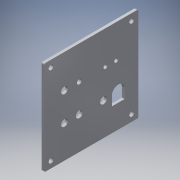
# Autodesk Inventor part: PP-LAS-0001
Saved by Autodesk Inventor 2018.3 (Build 223284000, 284)
## iProperties
Created: 2021-05-05
Part Number: PP-LAS-0001
Material: Plástico ABS
Document SubType Name: Modeling
Designer: L.Aguerre
Density: 1.06 g/cm^3
Appearance: Suave - Blanco
Description: FRENTE DE PANEL SERIGRAFIADO
Author: laguerre
Autodesk Inventor part; units mm, degrees
(part 1 of 3)
ref_plane "YZ Plane" through (0, 0, 0) normal (1, 0, 0) x (0, 1, 0)
ref_plane "XZ Plane" through (0, 0, 0) normal (0, 1, 0) x (-1, 0, 0)
ref_plane "XY Plane" through (0, 0, 0) normal (0, 0, 1) x (1, 0, 0)
sketch "Boceto39" plane through (0, 0, 0) normal (0, 0, 1) x (1, 0, 0)
  line L0 (-34, 35) -> (34, 35)
  line L1 (35, 34) -> (35, -34)
  line L2 (34, -35) -> (-34, -35)
  line L3 (-35, -34) -> (-35, 34)
  arc A0 (-34, 35) -> (-35, 34) centre (-34, 34) ccw
  arc A1 (35, 34) -> (34, 35) centre (34, 34) ccw
  arc A2 (34, -35) -> (35, -34) centre (34, -34) ccw
  arc A3 (-35, -34) -> (-34, -35) centre (-34, -34) ccw
  point P0 (0, 0)
  point P1 (0, 35)
  point P2 (-35, 0)
  dimension "d373" = 70
  dimension "d374" = 70
  dimension "d375" = 1
  constraints: 8 end point, 8 point on circle, 8 tangent, 4 centre point, 3 equal radius, 2 midpoint, 2 parallel, 1 horizontal, 1 horizontal alignment, 1 perpendicular, 1 vertical alignment
  measures "d373" distance between parallel lines of L1 L3
  measures "d374" distance between parallel lines of L2 L0
  measures "d375" radius of A0
extrude "Extrusión13" add sketch "Boceto39" along normal blind 2
sketch "Boceto43" plane through (0, 0, 2) normal (0, 0, 1) x (1, 0, 0)
  line L0 (-30, 30) -> (30, 30) construction
  line L1 (30, 30) -> (30, -30) construction
  line L2 (30, -30) -> (-30, -30) construction
  line L3 (-30, -30) -> (-30, 30) construction
  point P0 (0, 0)
  point P1 (0, 30)
  point P2 (-30, 0)
  dimension "d402" = 60
  constraints: 8 end point, 2 coincident, 2 midpoint, 2 parallel, 2 perpendicular, 1 horizontal, 1 horizontal alignment, 1 point on line, 1 vertical alignment
  measures "d402" distance of L0.start L0.end
hole "Agujero2" at (30, 30, 2) at (30, -30, 2) at (-30, -30, 2) at (-30, 30, 2) direction (0, 0, -1) diameter 3.5 depth 8 tip angle 118
sketch "Boceto40" plane through (0, 0, 2) normal (0, 0, 1) x (1, 0, 0)
  line L0 (-25, 0) -> (-4, 0)
  line L1 (-2, -2) -> (-2, -18)
  line L2 (-4, -20) -> (-25, -20)
  line L3 (-27, -18) -> (-27, -2)
  line L4 (4, 0) -> (25, 0)
  line L5 (27, -2) -> (27, -18)
  line L6 (25, -20) -> (4, -20)
  line L7 (2, -18) -> (2, -2)
  line L8 (-25, 20) -> (25, 20)
  line L9 (27, 18) -> (27, 5)
  line L10 (25, 3) -> (-25, 3)
  line L11 (-27, 5) -> (-27, 18)
  arc A0 (-27, -18) -> (-25, -20) centre (-25, -18) ccw
  arc A1 (-4, -20) -> (-2, -18) centre (-4, -18) ccw
  arc A2 (-2, -2) -> (-4, 0) centre (-4, -2) ccw
  arc A3 (-25, 0) -> (-27, -2) centre (-25, -2) ccw
  arc A4 (4, 0) -> (2, -2) centre (4, -2) ccw
  arc A5 (2, -18) -> (4, -20) centre (4, -18) ccw
  arc A6 (25, -20) -> (27, -18) centre (25, -18) ccw
  arc A7 (27, -2) -> (25, 0) centre (25, -2) ccw
  line L12 (-34, -35) -> (34, -35) projected
  arc A8 (-27, 5) -> (-25, 3) centre (-25, 5) ccw
  arc A9 (-25, 20) -> (-27, 18) centre (-25, 18) ccw
  arc A10 (27, 18) -> (25, 20) centre (25, 18) ccw
  arc A11 (25, 3) -> (27, 5) centre (25, 5) ccw
  line L13 (25, 19.7) -> (-25, 19.7)
  arc A12 (-25, 19.7) -> (-26.7, 18) centre (-25, 18) ccw
  line L14 (-26.7, 18) -> (-26.7, 5)
  arc A13 (-26.7, 5) -> (-25, 3.3) centre (-25, 5) ccw
  line L15 (-25, 3.3) -> (25, 3.3)
  arc A14 (25, 3.3) -> (26.7, 5) centre (25, 5) ccw
  line L16 (26.7, 5) -> (26.7, 18)
  arc A15 (26.7, 18) -> (25, 19.7) centre (25, 18) ccw
  line L17 (-4, -0.3) -> (-25, -0.3)
  arc A16 (-25, -0.3) -> (-26.7, -2) centre (-25, -2) ccw
  line L18 (-26.7, -2) -> (-26.7, -18)
  arc A17 (-26.7, -18) -> (-25, -19.7) centre (-25, -18) ccw
  line L19 (-25, -19.7) -> (-4, -19.7)
  arc A18 (-4, -19.7) -> (-2.3, -18) centre (-4, -18) ccw
  line L20 (-2.3, -18) -> (-2.3, -2)
  arc A19 (-2.3, -2) -> (-4, -0.3) centre (-4, -2) ccw
  line L21 (25, -0.3) -> (4, -0.3)
  arc A20 (4, -0.3) -> (2.3, -2) centre (4, -2) ccw
  line L22 (2.3, -2) -> (2.3, -18)
  arc A21 (2.3, -18) -> (4, -19.7) centre (4, -18) ccw
  line L23 (4, -19.7) -> (25, -19.7)
  arc A22 (25, -19.7) -> (26.7, -18) centre (25, -18) ccw
  line L24 (26.7, -18) -> (26.7, -2)
  arc A23 (26.7, -2) -> (25, -0.3) centre (25, -2) ccw
  point P0 (0, 0)
  point P1 (-27, 0)
  point P2 (-2, -20)
  point P3 (-27, -20)
  point P4 (27, -20)
  point P5 (2, -20)
  point P6 (0, 20)
  dimension "d378" = 2
  dimension "d379" = 2
  dimension "d380" = 25
  dimension "d381" = 25
  dimension "d382" = 20
  dimension "d383" = 2
  dimension "d385" = 3
  dimension "d386" = 2
  dimension "d387" = 17
  dimension "d388" = 0.3
  dimension "d389" = 0.3
  dimension "d390" = 0.3
  dimension "d477" = 20
  constraints: 48 end point, 48 point on circle, 24 centre point, 24 tangent, 12 parallel, 10 equal radius, 10 point on line, 6 perpendicular, 3 collinear, 3 horizontal, 1 midpoint, 1 vertical alignment, 21 other
  measures "d378" distance from line of point (0, 0) L1
  measures "d379" distance from line of point (0, 0) L7
  measures "d380" distance of point (-2, -20) point (-27, -20)
  measures "d381" distance of point (27, -20) point (2, -20)
  measures "d382" distance of point (-27, -20) point (-27, 0)
  measures "d383" radius of A0
  measures "d385" distance between parallel lines of L10 L0
  measures "d386" radius of A8
  measures "d387" distance between parallel lines of L8 L10
  measures "d388" distance between parallel lines of L15 L10
  measures "d389" distance between parallel lines of L4 L21
  measures "d390" distance between parallel lines of L0 L17
  measures "d477" distance from line of L6 point (0, 0)
extrude "Extrusión14" add sketch "Boceto40" along normal blind 0.001
sketch "Boceto41" plane through (0, 0, 2) normal (0, 0, 1) x (1, 0, 0)
  circle A0 centre (-20, -10.7) radius 5 construction
  line L0 (-34, -35) -> (34, -35) projected
  line L1 (-35, 34) -> (-35, -34) projected
  circle A1 centre (-9, -10.7) radius 2.5
  line L2 (-20, -10.7) -> (-9, -10.7) construction
  line L3 (-4, -19.7) -> (-25, -19.7) projected
  circle A2 centre (9, -10.7) radius 2.5
  circle A3 centre (20, -10.7) radius 2.5
  line L4 (25, -19.7) -> (4, -19.7) projected
  circle A4 centre (-18.5, 10.3) radius 1.5
  circle A5 centre (-10.5, 10.3) radius 1.5
  line L5 (-18.5, 10.3) -> (-10.5, 10.3) construction
  line L6 (25, 3.3) -> (-25, 3.3) projected
  circle A6 centre (20, 10.3) radius 2.5
  circle A7 centre (9, 10.3) radius 1.75
  line L7 (9, -10.7) -> (20, -10.7) construction
  line L8 (9, 10.3) -> (20, 10.3) construction
  line L9 (-24.7, -10.7) -> (-24.7, -17.7)
  line L10 (-24.7, -17.7) -> (-15.3, -17.7)
  line L11 (-15.3, -17.7) -> (-15.3, -10.7)
  arc A8 (-15.3, -10.7) -> (-24.7, -10.7) centre (-20, -10.7) ccw
  line L12 (-20, -6) -> (-22.9713, -6) construction
  point P0 (0, 0)
  point P1 (-14.5, -10.7)
  point P2 (-14.5, -19.7)
  point P3 (-14.5, 10.3)
  point P4 (14.5, -10.7)
  point P5 (14.5, -19.7)
  point P6 (14.5, 10.3)
  point P7 (-20, -17.7)
  dimension "d393" = 10
  dimension "d396" = 5
  dimension "d397" = 11
  dimension "d399" = 11
  dimension "d410" = 9
  dimension "d415" = 3
  dimension "d416" = 7
  dimension "d417" = 8
  dimension "d418" = 3.5
  dimension "d419" = 11
  dimension "d474" = 9.4
  dimension "d475" = 7
  dimension "d476" = 4.7
  constraints: 16 end point, 9 centre point, 7 midpoint, 5 horizontal, 5 horizontal alignment, 5 vertical alignment, 4 equal radius, 3 point on circle, 3 tangent, 2 perpendicular, 1 coincident, 1 vertical
  measures "d393" diameter of A0
  measures "d396" diameter of A1
  measures "d397" distance of L2.start L2.end
  measures "d399" distance of L7.end L7.start
  measures "d410" distance between parallel lines of L2 L3
  measures "d415" diameter of A5
  measures "d416" distance between parallel lines of L5 L6
  measures "d417" distance of L5.start L5.end
  measures "d418" diameter of A7
  measures "d419" distance of L8.end L8.start
  measures "d474" distance of L9.end L10.end
  measures "d475" distance from line of L2.start L10
  measures "d476" distance from line of L2.start L12
extrude "Extrusión15" cut sketch "Boceto41" against normal blind 2
sketch "Boceto42" plane through (0, 0, 2) normal (0, 0, 1) x (1, 0, 0)
  line L0 (-19.9009, -2.7) -> (-1.3327, -2.7) construction
  line L1 (-1.3327, -2.7) -> (-1.3327, -6.6561) construction
  line L2 (-1.3327, -6.6561) -> (-19.9009, -6.6561) construction
  line L3 (-19.9009, -6.6561) -> (-19.9009, -2.7) construction
  line L4 (-11.8025, -15.7) -> (-8.1255, -15.7) construction
  line L5 (-8.1255, -15.7) -> (-8.1255, -16.9024) construction
  line L6 (-8.1255, -16.9024) -> (-11.8025, -16.9024) construction
  line L7 (-11.8025, -16.9024) -> (-11.8025, -15.7) construction
  line L8 (6.4191, -2.7) -> (25.511, -2.7) construction
  line L9 (25.511, -2.7) -> (25.511, -5.9558) construction
  line L10 (25.511, -5.9558) -> (6.4191, -5.9558) construction
  line L11 (6.4191, -5.9558) -> (6.4191, -2.7) construction
  line L12 (7.0108, -15.7) -> (12.5482, -15.7) construction
  line L13 (12.5482, -15.7) -> (12.5482, -16.8686) construction
  line L14 (12.5482, -16.8686) -> (7.0108, -16.8686) construction
  line L15 (7.0108, -16.8686) -> (7.0108, -15.7) construction
  line L16 (17.6981, -15.7) -> (23.2355, -15.7) construction
  line L17 (23.2355, -15.7) -> (23.2355, -15.9466) construction
  line L18 (23.2355, -15.9466) -> (17.6981, -15.9466) construction
  line L19 (17.6981, -15.9466) -> (17.6981, -15.7) construction
  circle A0 centre (9, -10.7) radius 2.5 projected
  line L20 (-18.1999, 5.1784) -> (-18.1999, 6.3) construction
  line L21 (-18.1999, 6.3) -> (-6.5736, 6.3) construction
  line L22 (-6.5736, 6.3) -> (-6.5736, 5.1784) construction
  line L23 (-6.5736, 5.1784) -> (-18.1999, 5.1784) construction
  line L24 (6.4525, 5.7678) -> (6.4525, 6.3) construction
  line L25 (6.4525, 6.3) -> (10.1295, 6.3) construction
  line L26 (10.1295, 6.3) -> (10.1295, 5.7678) construction
  line L27 (10.1295, 5.7678) -> (6.4525, 5.7678) construction
  circle A1 centre (-18.5, 10.3) radius 1.5 projected
  line L28 (-22.5122, 16.6992) -> (-6.3487, 16.6992) construction
  line L29 (-6.3487, 16.6992) -> (-6.3487, 14.435) construction
  line L30 (-6.3487, 14.435) -> (-22.5122, 14.435) construction
  line L31 (-22.5122, 14.435) -> (-22.5122, 16.6992) construction
  line L32 (6.7652, 14.2645) -> (6.7652, 16.6992) construction
  line L33 (6.7652, 16.6992) -> (24.191, 16.6992) construction
  line L34 (24.191, 16.6992) -> (24.191, 14.2645) construction
  line L35 (24.191, 14.2645) -> (6.7652, 14.2645) construction
  line L36 (17.5924, 5.1479) -> (17.5924, 6.3) construction
  line L37 (17.5924, 6.3) -> (21.2695, 6.3) construction
  line L38 (21.2695, 6.3) -> (21.2695, 5.1479) construction
  line L39 (21.2695, 5.1479) -> (17.5924, 5.1479) construction
  line L40 (-19.0013, -4.7421) -> (-19.7761, -4.7421)
  line L41 (-19.7761, -4.7421) -> (-19.7761, -4.5379)
  line L42 (-19.7761, -4.5379) -> (-19.5216, -4.5379)
  line L43 (-19.5216, -4.5379) -> (-19.5216, -2.9464)
  line L44 (-19.5216, -2.9464) -> (-19.7761, -2.9464)
  line L45 (-19.7761, -2.9464) -> (-19.7761, -2.7421)
  line L46 (-19.7761, -2.7421) -> (-19.0013, -2.7421)
  line L47 (-19.0013, -2.7421) -> (-19.0013, -2.9464)
  line L48 (-19.0013, -2.9464) -> (-19.2558, -2.9464)
  line L49 (-19.2558, -2.9464) -> (-19.2558, -4.5379)
  line L50 (-19.2558, -4.5379) -> (-19.0013, -4.5379)
  line L51 (-19.0013, -4.5379) -> (-19.0013, -4.7421)
  line L52 (-17.2412, -4.7421) -> (-17.5394, -4.7421)
  line L53 (-17.5394, -4.7421) -> (-18.4244, -3.0177)
  line L54 (-18.4244, -3.0177) -> (-18.4244, -4.7421)
  line L55 (-18.4244, -4.7421) -> (-18.6723, -4.7421)
  line L56 (-18.6723, -4.7421) -> (-18.6723, -2.7421)
  line L57 (-18.6723, -2.7421) -> (-18.2947, -2.7421)
  line L58 (-18.2947, -2.7421) -> (-17.4892, -4.3256)
  line L59 (-17.4892, -4.3256) -> (-17.4892, -2.7421)
  line L60 (-17.4892, -2.7421) -> (-17.2412, -2.7421)
  line L61 (-17.2412, -2.7421) -> (-17.2412, -4.7421)
  spline S0 degree 2 poles (-15.5719, -3.3451) (-15.5719, -3.4747) (-15.6642, -3.7081) (-15.7469, -3.7891) knots 0 0 0 1 2 2 2
  spline S1 degree 2 poles (-15.7469, -3.7891) (-15.8506, -3.8912) (-16.131, -3.9966) (-16.3449, -3.9966) knots 0 0 0 1 2 2 2
  line L62 (-16.3449, -3.9966) -> (-16.5702, -3.9966)
  line L63 (-16.5702, -3.9966) -> (-16.5702, -4.7421)
  line L64 (-16.5702, -4.7421) -> (-16.836, -4.7421)
  line L65 (-16.836, -4.7421) -> (-16.836, -2.7421)
  line L66 (-16.836, -2.7421) -> (-16.3336, -2.7421)
  spline S2 degree 2 poles (-16.3336, -2.7421) (-16.1553, -2.7421) (-15.9057, -2.8005) (-15.8101, -2.8669) knots 0 0 0 1 2 2 2
  spline S3 degree 2 poles (-15.8101, -2.8669) (-15.6983, -2.9431) (-15.5719, -3.1781) (-15.5719, -3.3451) knots 0 0 0 1 2 2 2
  spline S4 degree 2 poles (-15.849, -3.3532) (-15.849, -3.2494) (-15.9203, -3.0971) (-15.9932, -3.0485) knots 0 0 0 1 2 2 2
  spline S5 degree 2 poles (-15.9932, -3.0485) (-16.0565, -3.0063) (-16.225, -2.9723) (-16.3498, -2.9723) knots 0 0 0 1 2 2 2
  line L67 (-16.3498, -2.9723) -> (-16.5702, -2.9723)
  line L68 (-16.5702, -2.9723) -> (-16.5702, -3.7697)
  line L69 (-16.5702, -3.7697) -> (-16.3887, -3.7697)
  spline S6 degree 2 poles (-16.3887, -3.7697) (-16.2266, -3.7697) (-16.0273, -3.7178) (-15.9625, -3.6498) knots 0 0 0 1 2 2 2
  spline S7 degree 2 poles (-15.9625, -3.6498) (-15.9025, -3.5898) (-15.849, -3.4488) (-15.849, -3.3532) knots 0 0 0 1 2 2 2
  spline S8 degree 2 poles (-14.6205, -4.7843) (-14.7971, -4.7843) (-15.0597, -4.6919) (-15.1521, -4.5995) knots 0 0 0 1 2 2 2
  spline S9 degree 2 poles (-15.1521, -4.5995) (-15.2574, -4.4958) (-15.3433, -4.2041) (-15.3433, -3.9901) knots 0 0 0 1 2 2 2
  line L70 (-15.3433, -3.9901) -> (-15.3433, -2.7421)
  line L71 (-15.3433, -2.7421) -> (-15.0775, -2.7421)
  line L72 (-15.0775, -2.7421) -> (-15.0775, -3.9901)
  spline S10 degree 2 poles (-15.0775, -3.9901) (-15.0775, -4.1295) (-15.0419, -4.3175) (-14.9916, -4.3937) knots 0 0 0 1 2 2 2
  spline S11 degree 2 poles (-14.9916, -4.3937) (-14.9381, -4.4747) (-14.7534, -4.5574) (-14.6205, -4.5574) knots 0 0 0 1 2 2 2
  spline S12 degree 2 poles (-14.6205, -4.5574) (-14.4957, -4.5574) (-14.3012, -4.4747) (-14.2477, -4.3937) knots 0 0 0 1 2 2 2
  spline S13 degree 2 poles (-14.2477, -4.3937) (-14.1975, -4.3175) (-14.1618, -4.1311) (-14.1618, -3.9966) knots 0 0 0 1 2 2 2
  line L73 (-14.1618, -3.9966) -> (-14.1618, -2.7421)
  line L74 (-14.1618, -2.7421) -> (-13.896, -2.7421)
  line L75 (-13.896, -2.7421) -> (-13.896, -3.9901)
  spline S14 degree 2 poles (-13.896, -3.9901) (-13.896, -4.1992) (-13.9803, -4.4974) (-14.0872, -4.5995) knots 0 0 0 1 2 2 2
  spline S15 degree 2 poles (-14.0872, -4.5995) (-14.1829, -4.6935) (-14.4357, -4.7843) (-14.6205, -4.7843) knots 0 0 0 1 2 2 2
  line L76 (-13.0484, -4.7421) -> (-13.0484, -2.9788)
  line L77 (-13.0484, -2.9788) -> (-13.7193, -2.9788)
  line L78 (-13.7193, -2.9788) -> (-13.7193, -2.7421)
  line L79 (-13.7193, -2.7421) -> (-12.1116, -2.7421)
  line L80 (-12.1116, -2.7421) -> (-12.1116, -2.9788)
  line L81 (-12.1116, -2.9788) -> (-12.7825, -2.9788)
  line L82 (-12.7825, -2.9788) -> (-12.7825, -4.7421)
  line L83 (-12.7825, -4.7421) -> (-13.0484, -4.7421)
  line L84 (-9.9738, -4.7421) -> (-10.9495, -4.7421)
  line L85 (-10.9495, -4.7421) -> (-10.9495, -4.5379)
  line L86 (-10.9495, -4.5379) -> (-10.5864, -4.5379)
  line L87 (-10.5864, -4.5379) -> (-10.5864, -3.1976)
  line L88 (-10.5864, -3.1976) -> (-10.9495, -3.1976)
  line L89 (-10.9495, -3.1976) -> (-10.9495, -3.0144)
  spline S16 degree 2 poles (-10.9495, -3.0144) (-10.7436, -3.0144) (-10.5492, -2.8977) (-10.5362, -2.7357) knots 0 0 0 1 2 2 2
  line L90 (-10.5362, -2.7357) -> (-10.3287, -2.7357)
  line L91 (-10.3287, -2.7357) -> (-10.3287, -4.5379)
  line L92 (-10.3287, -4.5379) -> (-9.9738, -4.5379)
  line L93 (-9.9738, -4.5379) -> (-9.9738, -4.7421)
  line L94 (-8.3725, -4.7421) -> (-9.6059, -4.7421)
  line L95 (-9.6059, -4.7421) -> (-9.6059, -4.4585)
  spline S17 degree 2 poles (-9.6059, -4.4585) (-9.473, -4.3337) (-9.2364, -4.1019) (-9.1229, -3.9771) knots 0 0 0 1 2 2 2
  spline S18 degree 2 poles (-9.1229, -3.9771) (-8.8944, -3.7259) (-8.7274, -3.4245) (-8.7274, -3.264) knots 0 0 0 1 2 2 2
  spline S19 degree 2 poles (-8.7274, -3.264) (-8.7274, -3.1797) (-8.7793, -3.0533) (-8.8263, -3.0128) knots 0 0 0 1 2 2 2
  spline S20 degree 2 poles (-8.8263, -3.0128) (-8.8733, -2.9723) (-8.9965, -2.9318) (-9.071, -2.9318) knots 0 0 0 1 2 2 2
  spline S21 degree 2 poles (-9.071, -2.9318) (-9.1424, -2.9318) (-9.2882, -2.9674) (-9.3547, -2.995) knots 0 0 0 1 2 2 2
  spline S22 degree 2 poles (-9.3547, -2.995) (-9.4114, -3.0177) (-9.5167, -3.0825) (-9.5492, -3.1052) knots 0 0 0 1 2 2 2
  line L96 (-9.5492, -3.1052) -> (-9.5637, -3.1052)
  line L97 (-9.5637, -3.1052) -> (-9.5637, -2.8199)
  spline S23 degree 2 poles (-9.5637, -2.8199) (-9.4811, -2.7794) (-9.1845, -2.7) (-9.0516, -2.7) knots 0 0 0 1 2 2 2
  spline S24 degree 2 poles (-9.0516, -2.7) (-8.7712, -2.7) (-8.4552, -2.9966) (-8.4552, -3.2494) knots 0 0 0 1 2 2 2
  spline S25 degree 2 poles (-8.4552, -3.2494) (-8.4552, -3.3677) (-8.5103, -3.5655) (-8.5589, -3.6498) knots 0 0 0 1 2 2 2
  spline S26 degree 2 poles (-8.5589, -3.6498) (-8.6075, -3.7373) (-8.7485, -3.9091) (-8.8263, -3.9917) knots 0 0 0 1 2 2 2
  spline S27 degree 2 poles (-8.8263, -3.9917) (-8.9527, -4.1295) (-9.2623, -4.4245) (-9.3547, -4.5104) knots 0 0 0 1 2 2 2
  line L98 (-9.3547, -4.5104) -> (-8.3725, -4.5104)
  line L99 (-8.3725, -4.5104) -> (-8.3725, -4.7421)
  line L100 (-6.5978, -2.7421) -> (-7.2866, -4.7421)
  line L101 (-7.2866, -4.7421) -> (-7.5735, -4.7421)
  line L102 (-7.5735, -4.7421) -> (-8.2623, -2.7421)
  line L103 (-8.2623, -2.7421) -> (-7.977, -2.7421)
  line L104 (-7.977, -2.7421) -> (-7.4227, -4.4034)
  line L105 (-7.4227, -4.4034) -> (-6.8684, -2.7421)
  line L106 (-6.8684, -2.7421) -> (-6.5978, -2.7421)
  spline S28 degree 2 poles (-10.7025, -16.1789) (-10.7025, -16.2762) (-10.7717, -16.4512) (-10.8337, -16.512) knots 0 0 0 1 2 2 2
  spline S29 degree 2 poles (-10.8337, -16.512) (-10.9115, -16.5886) (-11.1218, -16.6676) (-11.2823, -16.6676) knots 0 0 0 1 2 2 2
  line L107 (-11.2823, -16.6676) -> (-11.4512, -16.6676)
  line L108 (-11.4512, -16.6676) -> (-11.4512, -17.2267)
  line L109 (-11.4512, -17.2267) -> (-11.6506, -17.2267)
  line L110 (-11.6506, -17.2267) -> (-11.6506, -15.7267)
  line L111 (-11.6506, -15.7267) -> (-11.2738, -15.7267)
  spline S30 degree 2 poles (-11.2738, -15.7267) (-11.1401, -15.7267) (-10.9529, -15.7705) (-10.8811, -15.8203) knots 0 0 0 1 2 2 2
  spline S31 degree 2 poles (-10.8811, -15.8203) (-10.7973, -15.8775) (-10.7025, -16.0537) (-10.7025, -16.1789) knots 0 0 0 1 2 2 2
  spline S32 degree 2 poles (-10.9103, -16.185) (-10.9103, -16.1072) (-10.9638, -15.9929) (-11.0185, -15.9565) knots 0 0 0 1 2 2 2
  spline S33 degree 2 poles (-11.0185, -15.9565) (-11.0659, -15.9249) (-11.1923, -15.8994) (-11.2859, -15.8994) knots 0 0 0 1 2 2 2
  line L112 (-11.2859, -15.8994) -> (-11.4512, -15.8994)
  line L113 (-11.4512, -15.8994) -> (-11.4512, -16.4974)
  line L114 (-11.4512, -16.4974) -> (-11.3151, -16.4974)
  spline S34 degree 2 poles (-11.3151, -16.4974) (-11.1935, -16.4974) (-11.044, -16.4585) (-10.9954, -16.4075) knots 0 0 0 1 2 2 2
  spline S35 degree 2 poles (-10.9954, -16.4075) (-10.9504, -16.3625) (-10.9103, -16.2567) (-10.9103, -16.185) knots 0 0 0 1 2 2 2
  line L115 (-9.6437, -17.2267) -> (-10.5128, -17.2267)
  line L116 (-10.5128, -17.2267) -> (-10.5128, -15.7267)
  line L117 (-10.5128, -15.7267) -> (-10.3135, -15.7267)
  line L118 (-10.3135, -15.7267) -> (-10.3135, -17.0493)
  line L119 (-10.3135, -17.0493) -> (-9.6437, -17.0493)
  line L120 (-9.6437, -17.0493) -> (-9.6437, -17.2267)
  spline S36 degree 2 poles (-8.963, -17.2583) (-9.0955, -17.2583) (-9.2924, -17.1891) (-9.3617, -17.1198) knots 0 0 0 1 2 2 2
  spline S37 degree 2 poles (-9.3617, -17.1198) (-9.4407, -17.042) (-9.5051, -16.8232) (-9.5051, -16.6627) knots 0 0 0 1 2 2 2
  line L121 (-9.5051, -16.6627) -> (-9.5051, -15.7267)
  line L122 (-9.5051, -15.7267) -> (-9.3058, -15.7267)
  line L123 (-9.3058, -15.7267) -> (-9.3058, -16.6627)
  spline S38 degree 2 poles (-9.3058, -16.6627) (-9.3058, -16.7673) (-9.279, -16.9083) (-9.2414, -16.9654) knots 0 0 0 1 2 2 2
  spline S39 degree 2 poles (-9.2414, -16.9654) (-9.2012, -17.0262) (-9.0627, -17.0882) (-8.963, -17.0882) knots 0 0 0 1 2 2 2
  spline S40 degree 2 poles (-8.963, -17.0882) (-8.8694, -17.0882) (-8.7235, -17.0262) (-8.6834, -16.9654) knots 0 0 0 1 2 2 2
  spline S41 degree 2 poles (-8.6834, -16.9654) (-8.6457, -16.9083) (-8.619, -16.7685) (-8.619, -16.6676) knots 0 0 0 1 2 2 2
  line L124 (-8.619, -16.6676) -> (-8.619, -15.7267)
  line L125 (-8.619, -15.7267) -> (-8.4196, -15.7267)
  line L126 (-8.4196, -15.7267) -> (-8.4196, -16.6627)
  spline S42 degree 2 poles (-8.4196, -16.6627) (-8.4196, -16.8195) (-8.4828, -17.0432) (-8.5631, -17.1198) knots 0 0 0 1 2 2 2
  spline S43 degree 2 poles (-8.5631, -17.1198) (-8.6348, -17.1903) (-8.8244, -17.2583) (-8.963, -17.2583) knots 0 0 0 1 2 2 2
  spline S44 degree 2 poles (-7.5055, -17.2559) (-7.6648, -17.2559) (-7.9285, -17.1587) (-8.0234, -17.0602) knots 0 0 0 1 2 2 2
  spline S45 degree 2 poles (-8.0234, -17.0602) (-8.1182, -16.9605) (-8.2191, -16.6664) (-8.2191, -16.4755) knots 0 0 0 1 2 2 2
  spline S46 degree 2 poles (-8.2191, -16.4755) (-8.2191, -16.2944) (-8.117, -16.0075) (-8.0221, -15.9054) knots 0 0 0 1 2 2 2
  spline S47 degree 2 poles (-8.0221, -15.9054) (-7.931, -15.807) (-7.6636, -15.7) (-7.5043, -15.7) knots 0 0 0 1 2 2 2
  spline S48 degree 2 poles (-7.5043, -15.7) (-7.4277, -15.7) (-7.2892, -15.7219) (-7.226, -15.7413) knots 0 0 0 1 2 2 2
  spline S49 degree 2 poles (-7.226, -15.7413) (-7.1749, -15.7559) (-7.0509, -15.8094) (-7.0132, -15.8288) knots 0 0 0 1 2 2 2
  line L127 (-7.0132, -15.8288) -> (-7.0132, -16.0695)
  line L128 (-7.0132, -16.0695) -> (-7.0302, -16.0695)
  spline S50 degree 2 poles (-7.0302, -16.0695) (-7.0679, -16.0367) (-7.1469, -15.9771) (-7.2199, -15.9431) knots 0 0 0 1 2 2 2
  spline S51 degree 2 poles (-7.2199, -15.9431) (-7.2807, -15.9127) (-7.4375, -15.8726) (-7.5274, -15.8726) knots 0 0 0 1 2 2 2
  spline S52 degree 2 poles (-7.5274, -15.8726) (-7.7438, -15.8726) (-8.0112, -16.1984) (-8.0112, -16.4694) knots 0 0 0 1 2 2 2
  spline S53 degree 2 poles (-8.0112, -16.4694) (-8.0112, -16.6202) (-7.9407, -16.8463) (-7.8738, -16.9241) knots 0 0 0 1 2 2 2
  spline S54 degree 2 poles (-7.8738, -16.9241) (-7.8094, -17.0019) (-7.6271, -17.0833) (-7.5128, -17.0833) knots 0 0 0 1 2 2 2
  spline S55 degree 2 poles (-7.5128, -17.0833) (-7.429, -17.0833) (-7.2612, -17.059) (-7.2041, -17.0347) knots 0 0 0 1 2 2 2
  line L129 (-7.2041, -17.0347) -> (-7.2041, -16.6469)
  line L130 (-7.2041, -16.6469) -> (-7.5517, -16.6469)
  line L131 (-7.5517, -16.6469) -> (-7.5517, -16.4719)
  line L132 (-7.5517, -16.4719) -> (-7.0072, -16.4719)
  line L133 (-7.0072, -16.4719) -> (-7.0072, -17.1271)
  spline S56 degree 2 poles (-7.0072, -17.1271) (-7.0448, -17.1441) (-7.1737, -17.1964) (-7.2284, -17.2122) knots 0 0 0 1 2 2 2
  spline S57 degree 2 poles (-7.2284, -17.2122) (-7.3025, -17.234) (-7.4217, -17.2559) (-7.5055, -17.2559) knots 0 0 0 1 2 2 2
  spline S58 degree 2 poles (-6.1283, -17.2559) (-6.2875, -17.2559) (-6.5513, -17.1587) (-6.6461, -17.0602) knots 0 0 0 1 2 2 2
  spline S59 degree 2 poles (-6.6461, -17.0602) (-6.7409, -16.9605) (-6.8418, -16.6664) (-6.8418, -16.4755) knots 0 0 0 1 2 2 2
  spline S60 degree 2 poles (-6.8418, -16.4755) (-6.8418, -16.2944) (-6.7397, -16.0075) (-6.6449, -15.9054) knots 0 0 0 1 2 2 2
  spline S61 degree 2 poles (-6.6449, -15.9054) (-6.5537, -15.807) (-6.2863, -15.7) (-6.1271, -15.7) knots 0 0 0 1 2 2 2
  spline S62 degree 2 poles (-6.1271, -15.7) (-6.0505, -15.7) (-5.9119, -15.7219) (-5.8487, -15.7413) knots 0 0 0 1 2 2 2
  spline S63 degree 2 poles (-5.8487, -15.7413) (-5.7977, -15.7559) (-5.6737, -15.8094) (-5.636, -15.8288) knots 0 0 0 1 2 2 2
  line L134 (-5.636, -15.8288) -> (-5.636, -16.0695)
  line L135 (-5.636, -16.0695) -> (-5.653, -16.0695)
  spline S64 degree 2 poles (-5.653, -16.0695) (-5.6907, -16.0367) (-5.7697, -15.9771) (-5.8426, -15.9431) knots 0 0 0 1 2 2 2
  spline S65 degree 2 poles (-5.8426, -15.9431) (-5.9034, -15.9127) (-6.0602, -15.8726) (-6.1502, -15.8726) knots 0 0 0 1 2 2 2
  spline S66 degree 2 poles (-6.1502, -15.8726) (-6.3666, -15.8726) (-6.634, -16.1984) (-6.634, -16.4694) knots 0 0 0 1 2 2 2
  spline S67 degree 2 poles (-6.634, -16.4694) (-6.634, -16.6202) (-6.5635, -16.8463) (-6.4966, -16.9241) knots 0 0 0 1 2 2 2
  spline S68 degree 2 poles (-6.4966, -16.9241) (-6.4322, -17.0019) (-6.2499, -17.0833) (-6.1356, -17.0833) knots 0 0 0 1 2 2 2
  spline S69 degree 2 poles (-6.1356, -17.0833) (-6.0517, -17.0833) (-5.884, -17.059) (-5.8268, -17.0347) knots 0 0 0 1 2 2 2
  line L136 (-5.8268, -17.0347) -> (-5.8268, -16.6469)
  line L137 (-5.8268, -16.6469) -> (-6.1745, -16.6469)
  line L138 (-6.1745, -16.6469) -> (-6.1745, -16.4719)
  line L139 (-6.1745, -16.4719) -> (-5.6299, -16.4719)
  line L140 (-5.6299, -16.4719) -> (-5.6299, -17.1271)
  spline S70 degree 2 poles (-5.6299, -17.1271) (-5.6676, -17.1441) (-5.7965, -17.1964) (-5.8512, -17.2122) knots 0 0 0 1 2 2 2
  spline S71 degree 2 poles (-5.8512, -17.2122) (-5.9253, -17.234) (-6.0444, -17.2559) (-6.1283, -17.2559) knots 0 0 0 1 2 2 2
  line L141 (-5.3795, -17.2267) -> (-5.3795, -15.7267)
  line L142 (-5.3795, -15.7267) -> (-4.4411, -15.7267)
  line L143 (-4.4411, -15.7267) -> (-4.4411, -15.9042)
  line L144 (-4.4411, -15.9042) -> (-5.1802, -15.9042)
  line L145 (-5.1802, -15.9042) -> (-5.1802, -16.3151)
  line L146 (-5.1802, -16.3151) -> (-4.4909, -16.3151)
  line L147 (-4.4909, -16.3151) -> (-4.4909, -16.4925)
  line L148 (-4.4909, -16.4925) -> (-5.1802, -16.4925)
  line L149 (-5.1802, -16.4925) -> (-5.1802, -17.0493)
  line L150 (-5.1802, -17.0493) -> (-4.4411, -17.0493)
  line L151 (-4.4411, -17.0493) -> (-4.4411, -17.2267)
  line L152 (-4.4411, -17.2267) -> (-5.3795, -17.2267)
  spline S72 degree 2 poles (-3.0396, -16.478) (-3.0396, -16.6834) (-3.2061, -17.014) (-3.3459, -17.1064) knots 0 0 0 1 2 2 2
  spline S73 degree 2 poles (-3.3459, -17.1064) (-3.4602, -17.1781) (-3.6948, -17.2267) (-3.8771, -17.2267) knots 0 0 0 1 2 2 2
  line L153 (-3.8771, -17.2267) -> (-4.2223, -17.2267)
  line L154 (-4.2223, -17.2267) -> (-4.2223, -15.7267)
  line L155 (-4.2223, -15.7267) -> (-3.8807, -15.7267)
  spline S74 degree 2 poles (-3.8807, -15.7267) (-3.6692, -15.7267) (-3.4285, -15.79) (-3.3435, -15.8459) knots 0 0 0 1 2 2 2
  spline S75 degree 2 poles (-3.3435, -15.8459) (-3.1988, -15.9419) (-3.0396, -16.2592) (-3.0396, -16.478) knots 0 0 0 1 2 2 2
  spline S76 degree 2 poles (-3.2474, -16.4755) (-3.2474, -16.3029) (-3.3617, -16.0586) (-3.4747, -15.9893) knots 0 0 0 1 2 2 2
  spline S77 degree 2 poles (-3.4747, -15.9893) (-3.555, -15.9419) (-3.7361, -15.8994) (-3.871, -15.8994) knots 0 0 0 1 2 2 2
  line L156 (-3.871, -15.8994) -> (-4.023, -15.8994)
  line L157 (-4.023, -15.8994) -> (-4.023, -17.0541)
  line L158 (-4.023, -17.0541) -> (-3.871, -17.0541)
  spline S78 degree 2 poles (-3.871, -17.0541) (-3.7385, -17.0541) (-3.5379, -17.0116) (-3.4565, -16.9545) knots 0 0 0 1 2 2 2
  spline S79 degree 2 poles (-3.4565, -16.9545) (-3.352, -16.884) (-3.2474, -16.6506) (-3.2474, -16.4755) knots 0 0 0 1 2 2 2
  line L159 (7.0884, -4.7357) -> (7.0884, -2.9723)
  line L160 (7.0884, -2.9723) -> (6.4174, -2.9723)
  line L161 (6.4174, -2.9723) -> (6.4174, -2.7357)
  line L162 (6.4174, -2.7357) -> (8.0252, -2.7357)
  line L163 (8.0252, -2.7357) -> (8.0252, -2.9723)
  line L164 (8.0252, -2.9723) -> (7.3542, -2.9723)
  line L165 (7.3542, -2.9723) -> (7.3542, -4.7357)
  line L166 (7.3542, -4.7357) -> (7.0884, -4.7357)
  line L167 (8.2278, -4.7357) -> (8.2278, -2.7357)
  line L168 (8.2278, -2.7357) -> (9.479, -2.7357)
  line L169 (9.479, -2.7357) -> (9.479, -2.9723)
  line L170 (9.479, -2.9723) -> (8.4936, -2.9723)
  line L171 (8.4936, -2.9723) -> (8.4936, -3.5201)
  line L172 (8.4936, -3.5201) -> (9.4126, -3.5201)
  line L173 (9.4126, -3.5201) -> (9.4126, -3.7567)
  line L174 (9.4126, -3.7567) -> (8.4936, -3.7567)
  line L175 (8.4936, -3.7567) -> (8.4936, -4.499)
  line L176 (8.4936, -4.499) -> (9.479, -4.499)
  line L177 (9.479, -4.499) -> (9.479, -4.7357)
  line L178 (9.479, -4.7357) -> (8.2278, -4.7357)
  spline S80 degree 2 poles (10.3283, -4.7713) (10.1111, -4.7713) (9.8064, -4.6806) (9.6719, -4.6157) knots 0 0 0 1 2 2 2
  line L179 (9.6719, -4.6157) -> (9.6719, -4.2818)
  line L180 (9.6719, -4.2818) -> (9.6913, -4.2818)
  spline S81 degree 2 poles (9.6913, -4.2818) (9.8226, -4.405) (10.1549, -4.5412) (10.3088, -4.5412) knots 0 0 0 1 2 2 2
  spline S82 degree 2 poles (10.3088, -4.5412) (10.5293, -4.5412) (10.7545, -4.358) (10.7545, -4.2073) knots 0 0 0 1 2 2 2
  spline S83 degree 2 poles (10.7545, -4.2073) (10.7545, -4.0874) (10.6362, -3.9382) (10.5082, -3.901) knots 0 0 0 1 2 2 2
  spline S84 degree 2 poles (10.5082, -3.901) (10.4158, -3.875) (10.2618, -3.8394) (10.1468, -3.8102) knots 0 0 0 1 2 2 2
  spline S85 degree 2 poles (10.1468, -3.8102) (10.043, -3.7827) (9.8793, -3.7) (9.8161, -3.6335) knots 0 0 0 1 2 2 2
  spline S86 degree 2 poles (9.8161, -3.6335) (9.7545, -3.5671) (9.6865, -3.3888) (9.6865, -3.2721) knots 0 0 0 1 2 2 2
  spline S87 degree 2 poles (9.6865, -3.2721) (9.6865, -3.029) (10.0657, -2.7) (10.3591, -2.7) knots 0 0 0 1 2 2 2
  spline S88 degree 2 poles (10.3591, -2.7) (10.5276, -2.7) (10.8259, -2.7665) (10.9539, -2.8297) knots 0 0 0 1 2 2 2
  line L181 (10.9539, -2.8297) -> (10.9539, -3.1473)
  line L182 (10.9539, -3.1473) -> (10.9344, -3.1473)
  spline S89 degree 2 poles (10.9344, -3.1473) (10.8388, -3.0598) (10.5406, -2.9301) (10.3769, -2.9301) knots 0 0 0 1 2 2 2
  spline S90 degree 2 poles (10.3769, -2.9301) (10.1921, -2.9301) (9.9636, -3.1036) (9.9636, -3.2446) knots 0 0 0 1 2 2 2
  spline S91 degree 2 poles (9.9636, -3.2446) (9.9636, -3.371) (10.0981, -3.5217) (10.2246, -3.5558) knots 0 0 0 1 2 2 2
  spline S92 degree 2 poles (10.2246, -3.5558) (10.3088, -3.5784) (10.5536, -3.6368) (10.6346, -3.6611) knots 0 0 0 1 2 2 2
  spline S93 degree 2 poles (10.6346, -3.6611) (10.8404, -3.7243) (11.0317, -3.9788) (11.0317, -4.1652) knots 0 0 0 1 2 2 2
  spline S94 degree 2 poles (11.0317, -4.1652) (11.0317, -4.2835) (10.9361, -4.5104) (10.8502, -4.5898) knots 0 0 0 1 2 2 2
  spline S95 degree 2 poles (10.8502, -4.5898) (10.7545, -4.6773) (10.5114, -4.7713) (10.3283, -4.7713) knots 0 0 0 1 2 2 2
  line L183 (11.7691, -4.7357) -> (11.7691, -2.9723)
  line L184 (11.7691, -2.9723) -> (11.0981, -2.9723)
  line L185 (11.0981, -2.9723) -> (11.0981, -2.7357)
  line L186 (11.0981, -2.7357) -> (12.7059, -2.7357)
  line L187 (12.7059, -2.7357) -> (12.7059, -2.9723)
  line L188 (12.7059, -2.9723) -> (12.0349, -2.9723)
  line L189 (12.0349, -2.9723) -> (12.0349, -4.7357)
  line L190 (12.0349, -4.7357) -> (11.7691, -4.7357)
  line L191 (15.3153, -4.7357) -> (14.9701, -4.7357)
  line L192 (14.9701, -4.7357) -> (14.338, -3.9399)
  line L193 (14.338, -3.9399) -> (14.0333, -3.9399)
  line L194 (14.0333, -3.9399) -> (14.0333, -4.7357)
  line L195 (14.0333, -4.7357) -> (13.7675, -4.7357)
  line L196 (13.7675, -4.7357) -> (13.7675, -2.7357)
  line L197 (13.7675, -2.7357) -> (14.2829, -2.7357)
  spline S96 degree 2 poles (14.2829, -2.7357) (14.4547, -2.7357) (14.6865, -2.7729) (14.7918, -2.841) knots 0 0 0 1 2 2 2
  spline S97 degree 2 poles (14.7918, -2.841) (14.8972, -2.9091) (15.0187, -3.1214) (15.0187, -3.2786) knots 0 0 0 1 2 2 2
  spline S98 degree 2 poles (15.0187, -3.2786) (15.0187, -3.4974) (14.7951, -3.794) (14.6038, -3.8653) knots 0 0 0 1 2 2 2
  line L198 (14.6038, -3.8653) -> (15.3153, -4.7357)
  spline S99 degree 2 poles (14.7416, -3.2997) (14.7416, -3.2122) (14.68, -3.0776) (14.6152, -3.0339) knots 0 0 0 1 2 2 2
  spline S100 degree 2 poles (14.6152, -3.0339) (14.5584, -2.9966) (14.4077, -2.9658) (14.2975, -2.9658) knots 0 0 0 1 2 2 2
  line L199 (14.2975, -2.9658) -> (14.0333, -2.9658)
  line L200 (14.0333, -2.9658) -> (14.0333, -3.7178)
  line L201 (14.0333, -3.7178) -> (14.2667, -3.7178)
  spline S101 degree 2 poles (14.2667, -3.7178) (14.3818, -3.7178) (14.5649, -3.6773) (14.6281, -3.6141) knots 0 0 0 1 2 2 2
  spline S102 degree 2 poles (14.6281, -3.6141) (14.6865, -3.559) (14.7416, -3.4034) (14.7416, -3.2997) knots 0 0 0 1 2 2 2
  line L202 (15.4742, -4.7357) -> (15.4742, -2.7357)
  line L203 (15.4742, -2.7357) -> (16.7254, -2.7357)
  line L204 (16.7254, -2.7357) -> (16.7254, -2.9723)
  line L205 (16.7254, -2.9723) -> (15.74, -2.9723)
  line L206 (15.74, -2.9723) -> (15.74, -3.5201)
  line L207 (15.74, -3.5201) -> (16.6589, -3.5201)
  line L208 (16.6589, -3.5201) -> (16.6589, -3.7567)
  line L209 (16.6589, -3.7567) -> (15.74, -3.7567)
  line L210 (15.74, -3.7567) -> (15.74, -4.499)
  line L211 (15.74, -4.499) -> (16.7254, -4.499)
  line L212 (16.7254, -4.499) -> (16.7254, -4.7357)
  line L213 (16.7254, -4.7357) -> (15.4742, -4.7357)
  spline S103 degree 2 poles (17.5746, -4.7713) (17.3575, -4.7713) (17.0528, -4.6806) (16.9182, -4.6157) knots 0 0 0 1 2 2 2
  line L214 (16.9182, -4.6157) -> (16.9182, -4.2818)
  line L215 (16.9182, -4.2818) -> (16.9377, -4.2818)
  spline S104 degree 2 poles (16.9377, -4.2818) (17.069, -4.405) (17.4012, -4.5412) (17.5552, -4.5412) knots 0 0 0 1 2 2 2
  spline S105 degree 2 poles (17.5552, -4.5412) (17.7756, -4.5412) (18.0009, -4.358) (18.0009, -4.2073) knots 0 0 0 1 2 2 2
  spline S106 degree 2 poles (18.0009, -4.2073) (18.0009, -4.0874) (17.8826, -3.9382) (17.7545, -3.901) knots 0 0 0 1 2 2 2
  spline S107 degree 2 poles (17.7545, -3.901) (17.6622, -3.875) (17.5082, -3.8394) (17.3931, -3.8102) knots 0 0 0 1 2 2 2
  spline S108 degree 2 poles (17.3931, -3.8102) (17.2894, -3.7827) (17.1257, -3.7) (17.0625, -3.6335) knots 0 0 0 1 2 2 2
  spline S109 degree 2 poles (17.0625, -3.6335) (17.0009, -3.5671) (16.9328, -3.3888) (16.9328, -3.2721) knots 0 0 0 1 2 2 2
  spline S110 degree 2 poles (16.9328, -3.2721) (16.9328, -3.029) (17.3121, -2.7) (17.6054, -2.7) knots 0 0 0 1 2 2 2
  spline S111 degree 2 poles (17.6054, -2.7) (17.774, -2.7) (18.0722, -2.7665) (18.2003, -2.8297) knots 0 0 0 1 2 2 2
  line L216 (18.2003, -2.8297) -> (18.2003, -3.1473)
  line L217 (18.2003, -3.1473) -> (18.1808, -3.1473)
  spline S112 degree 2 poles (18.1808, -3.1473) (18.0852, -3.0598) (17.787, -2.9301) (17.6233, -2.9301) knots 0 0 0 1 2 2 2
  spline S113 degree 2 poles (17.6233, -2.9301) (17.4385, -2.9301) (17.21, -3.1036) (17.21, -3.2446) knots 0 0 0 1 2 2 2
  spline S114 degree 2 poles (17.21, -3.2446) (17.21, -3.371) (17.3445, -3.5217) (17.4709, -3.5558) knots 0 0 0 1 2 2 2
  spline S115 degree 2 poles (17.4709, -3.5558) (17.5552, -3.5784) (17.7999, -3.6368) (17.881, -3.6611) knots 0 0 0 1 2 2 2
  spline S116 degree 2 poles (17.881, -3.6611) (18.0868, -3.7243) (18.278, -3.9788) (18.278, -4.1652) knots 0 0 0 1 2 2 2
  spline S117 degree 2 poles (18.278, -4.1652) (18.278, -4.2835) (18.1824, -4.5104) (18.0965, -4.5898) knots 0 0 0 1 2 2 2
  spline S118 degree 2 poles (18.0965, -4.5898) (18.0009, -4.6773) (17.7578, -4.7713) (17.5746, -4.7713) knots 0 0 0 1 2 2 2
  spline S119 degree 2 poles (19.2473, -4.7778) (19.0706, -4.7778) (18.808, -4.6854) (18.7156, -4.593) knots 0 0 0 1 2 2 2
  spline S120 degree 2 poles (18.7156, -4.593) (18.6103, -4.4893) (18.5244, -4.1976) (18.5244, -3.9836) knots 0 0 0 1 2 2 2
  line L218 (18.5244, -3.9836) -> (18.5244, -2.7357)
  line L219 (18.5244, -2.7357) -> (18.7902, -2.7357)
  line L220 (18.7902, -2.7357) -> (18.7902, -3.9836)
  spline S121 degree 2 poles (18.7902, -3.9836) (18.7902, -4.123) (18.8259, -4.311) (18.8761, -4.3872) knots 0 0 0 1 2 2 2
  spline S122 degree 2 poles (18.8761, -4.3872) (18.9296, -4.4682) (19.1144, -4.5509) (19.2473, -4.5509) knots 0 0 0 1 2 2 2
  spline S123 degree 2 poles (19.2473, -4.5509) (19.372, -4.5509) (19.5665, -4.4682) (19.62, -4.3872) knots 0 0 0 1 2 2 2
  spline S124 degree 2 poles (19.62, -4.3872) (19.6703, -4.311) (19.7059, -4.1246) (19.7059, -3.9901) knots 0 0 0 1 2 2 2
  line L221 (19.7059, -3.9901) -> (19.7059, -2.7357)
  line L222 (19.7059, -2.7357) -> (19.9717, -2.7357)
  line L223 (19.9717, -2.7357) -> (19.9717, -3.9836)
  spline S125 degree 2 poles (19.9717, -3.9836) (19.9717, -4.1927) (19.8874, -4.4909) (19.7805, -4.593) knots 0 0 0 1 2 2 2
  spline S126 degree 2 poles (19.7805, -4.593) (19.6849, -4.687) (19.432, -4.7778) (19.2473, -4.7778) knots 0 0 0 1 2 2 2
  line L224 (21.5114, -4.7357) -> (20.3526, -4.7357)
  line L225 (20.3526, -4.7357) -> (20.3526, -2.7357)
  line L226 (20.3526, -2.7357) -> (20.6184, -2.7357)
  line L227 (20.6184, -2.7357) -> (20.6184, -4.499)
  line L228 (20.6184, -4.499) -> (21.5114, -4.499)
  line L229 (21.5114, -4.499) -> (21.5114, -4.7357)
  line L230 (22.1873, -4.7357) -> (22.1873, -2.9723)
  line L231 (22.1873, -2.9723) -> (21.5163, -2.9723)
  line L232 (21.5163, -2.9723) -> (21.5163, -2.7357)
  line L233 (21.5163, -2.7357) -> (23.1241, -2.7357)
  line L234 (23.1241, -2.7357) -> (23.1241, -2.9723)
  line L235 (23.1241, -2.9723) -> (22.4531, -2.9723)
  line L236 (22.4531, -2.9723) -> (22.4531, -4.7357)
  line L237 (22.4531, -4.7357) -> (22.1873, -4.7357)
  spline S127 degree 2 poles (23.8842, -4.7713) (23.667, -4.7713) (23.3623, -4.6806) (23.2278, -4.6157) knots 0 0 0 1 2 2 2
  line L238 (23.2278, -4.6157) -> (23.2278, -4.2818)
  line L239 (23.2278, -4.2818) -> (23.2473, -4.2818)
  spline S128 degree 2 poles (23.2473, -4.2818) (23.3785, -4.405) (23.7108, -4.5412) (23.8648, -4.5412) knots 0 0 0 1 2 2 2
  spline S129 degree 2 poles (23.8648, -4.5412) (24.0852, -4.5412) (24.3105, -4.358) (24.3105, -4.2073) knots 0 0 0 1 2 2 2
  spline S130 degree 2 poles (24.3105, -4.2073) (24.3105, -4.0874) (24.1921, -3.9382) (24.0641, -3.901) knots 0 0 0 1 2 2 2
  spline S131 degree 2 poles (24.0641, -3.901) (23.9717, -3.875) (23.8178, -3.8394) (23.7027, -3.8102) knots 0 0 0 1 2 2 2
  spline S132 degree 2 poles (23.7027, -3.8102) (23.599, -3.7827) (23.4353, -3.7) (23.372, -3.6335) knots 0 0 0 1 2 2 2
  spline S133 degree 2 poles (23.372, -3.6335) (23.3105, -3.5671) (23.2424, -3.3888) (23.2424, -3.2721) knots 0 0 0 1 2 2 2
  spline S134 degree 2 poles (23.2424, -3.2721) (23.2424, -3.029) (23.6216, -2.7) (23.915, -2.7) knots 0 0 0 1 2 2 2
  spline S135 degree 2 poles (23.915, -2.7) (24.0836, -2.7) (24.3818, -2.7665) (24.5098, -2.8297) knots 0 0 0 1 2 2 2
  line L240 (24.5098, -2.8297) -> (24.5098, -3.1473)
  line L241 (24.5098, -3.1473) -> (24.4904, -3.1473)
  spline S136 degree 2 poles (24.4904, -3.1473) (24.3947, -3.0598) (24.0965, -2.9301) (23.9328, -2.9301) knots 0 0 0 1 2 2 2
  spline S137 degree 2 poles (23.9328, -2.9301) (23.7481, -2.9301) (23.5195, -3.1036) (23.5195, -3.2446) knots 0 0 0 1 2 2 2
  spline S138 degree 2 poles (23.5195, -3.2446) (23.5195, -3.371) (23.6541, -3.5217) (23.7805, -3.5558) knots 0 0 0 1 2 2 2
  spline S139 degree 2 poles (23.7805, -3.5558) (23.8648, -3.5784) (24.1095, -3.6368) (24.1905, -3.6611) knots 0 0 0 1 2 2 2
  spline S140 degree 2 poles (24.1905, -3.6611) (24.3964, -3.7243) (24.5876, -3.9788) (24.5876, -4.1652) knots 0 0 0 1 2 2 2
  spline S141 degree 2 poles (24.5876, -4.1652) (24.5876, -4.2835) (24.492, -4.5104) (24.4061, -4.5898) knots 0 0 0 1 2 2 2
  spline S142 degree 2 poles (24.4061, -4.5898) (24.3105, -4.6773) (24.0673, -4.7713) (23.8842, -4.7713) knots 0 0 0 1 2 2 2
  spline S143 degree 2 poles (18.7982, -16.1789) (18.7982, -16.2762) (18.7289, -16.4512) (18.6669, -16.512) knots 0 0 0 1 2 2 2
  spline S144 degree 2 poles (18.6669, -16.512) (18.5891, -16.5886) (18.3788, -16.6676) (18.2183, -16.6676) knots 0 0 0 1 2 2 2
  line L242 (18.2183, -16.6676) -> (18.0494, -16.6676)
  line L243 (18.0494, -16.6676) -> (18.0494, -17.2267)
  line L244 (18.0494, -17.2267) -> (17.85, -17.2267)
  line L245 (17.85, -17.2267) -> (17.85, -15.7267)
  line L246 (17.85, -15.7267) -> (18.2268, -15.7267)
  spline S145 degree 2 poles (18.2268, -15.7267) (18.3606, -15.7267) (18.5477, -15.7705) (18.6195, -15.8203) knots 0 0 0 1 2 2 2
  spline S146 degree 2 poles (18.6195, -15.8203) (18.7033, -15.8775) (18.7982, -16.0537) (18.7982, -16.1789) knots 0 0 0 1 2 2 2
  spline S147 degree 2 poles (18.5903, -16.185) (18.5903, -16.1072) (18.5368, -15.9929) (18.4821, -15.9565) knots 0 0 0 1 2 2 2
  spline S148 degree 2 poles (18.4821, -15.9565) (18.4347, -15.9249) (18.3083, -15.8994) (18.2147, -15.8994) knots 0 0 0 1 2 2 2
  line L247 (18.2147, -15.8994) -> (18.0494, -15.8994)
  line L248 (18.0494, -15.8994) -> (18.0494, -16.4974)
  line L249 (18.0494, -16.4974) -> (18.1855, -16.4974)
  spline S149 degree 2 poles (18.1855, -16.4974) (18.3071, -16.4974) (18.4566, -16.4585) (18.5052, -16.4075) knots 0 0 0 1 2 2 2
  spline S150 degree 2 poles (18.5052, -16.4075) (18.5502, -16.3625) (18.5903, -16.2567) (18.5903, -16.185) knots 0 0 0 1 2 2 2
  line L250 (18.8261, -17.2267) -> (19.3318, -15.7267)
  line L251 (19.3318, -15.7267) -> (19.5773, -15.7267)
  line L252 (19.5773, -15.7267) -> (20.083, -17.2267)
  line L253 (20.083, -17.2267) -> (19.8727, -17.2267)
  line L254 (19.8727, -17.2267) -> (19.7366, -16.8074)
  line L255 (19.7366, -16.8074) -> (19.164, -16.8074)
  line L256 (19.164, -16.8074) -> (19.0279, -17.2267)
  line L257 (19.0279, -17.2267) -> (18.8261, -17.2267)
  line L258 (19.6819, -16.6372) -> (19.4497, -15.931)
  line L259 (19.4497, -15.931) -> (19.2187, -16.6372)
  line L260 (19.2187, -16.6372) -> (19.6819, -16.6372)
  spline S151 degree 2 poles (20.6434, -17.2535) (20.4805, -17.2535) (20.252, -17.1854) (20.1511, -17.1368) knots 0 0 0 1 2 2 2
  line L261 (20.1511, -17.1368) -> (20.1511, -16.8864)
  line L262 (20.1511, -16.8864) -> (20.1657, -16.8864)
  spline S152 degree 2 poles (20.1657, -16.8864) (20.2641, -16.9788) (20.5133, -17.0809) (20.6288, -17.0809) knots 0 0 0 1 2 2 2
  spline S153 degree 2 poles (20.6288, -17.0809) (20.7941, -17.0809) (20.9631, -16.9435) (20.9631, -16.8305) knots 0 0 0 1 2 2 2
  spline S154 degree 2 poles (20.9631, -16.8305) (20.9631, -16.7405) (20.8743, -16.6287) (20.7783, -16.6007) knots 0 0 0 1 2 2 2
  spline S155 degree 2 poles (20.7783, -16.6007) (20.709, -16.5813) (20.5935, -16.5545) (20.5072, -16.5327) knots 0 0 0 1 2 2 2
  spline S156 degree 2 poles (20.5072, -16.5327) (20.4294, -16.512) (20.3067, -16.45) (20.2593, -16.4002) knots 0 0 0 1 2 2 2
  spline S157 degree 2 poles (20.2593, -16.4002) (20.2131, -16.3503) (20.162, -16.2166) (20.162, -16.1291) knots 0 0 0 1 2 2 2
  spline S158 degree 2 poles (20.162, -16.1291) (20.162, -15.9468) (20.4465, -15.7) (20.6665, -15.7) knots 0 0 0 1 2 2 2
  spline S159 degree 2 poles (20.6665, -15.7) (20.7929, -15.7) (21.0165, -15.7498) (21.1126, -15.7972) knots 0 0 0 1 2 2 2
  line L263 (21.1126, -15.7972) -> (21.1126, -16.0355)
  line L264 (21.1126, -16.0355) -> (21.098, -16.0355)
  spline S160 degree 2 poles (21.098, -16.0355) (21.0263, -15.9699) (20.8026, -15.8726) (20.6798, -15.8726) knots 0 0 0 1 2 2 2
  spline S161 degree 2 poles (20.6798, -15.8726) (20.5413, -15.8726) (20.3699, -16.0027) (20.3699, -16.1084) knots 0 0 0 1 2 2 2
  spline S162 degree 2 poles (20.3699, -16.1084) (20.3699, -16.2032) (20.4708, -16.3163) (20.5656, -16.3418) knots 0 0 0 1 2 2 2
  spline S163 degree 2 poles (20.5656, -16.3418) (20.6288, -16.3588) (20.8123, -16.4026) (20.8731, -16.4208) knots 0 0 0 1 2 2 2
  spline S164 degree 2 poles (20.8731, -16.4208) (21.0275, -16.4682) (21.1709, -16.6591) (21.1709, -16.7989) knots 0 0 0 1 2 2 2
  spline S165 degree 2 poles (21.1709, -16.7989) (21.1709, -16.8876) (21.0992, -17.0578) (21.0348, -17.1173) knots 0 0 0 1 2 2 2
  spline S166 degree 2 poles (21.0348, -17.1173) (20.9631, -17.183) (20.7807, -17.2535) (20.6434, -17.2535) knots 0 0 0 1 2 2 2
  spline S167 degree 2 poles (21.7921, -17.2535) (21.6292, -17.2535) (21.4007, -17.1854) (21.2998, -17.1368) knots 0 0 0 1 2 2 2
  line L265 (21.2998, -17.1368) -> (21.2998, -16.8864)
  line L266 (21.2998, -16.8864) -> (21.3144, -16.8864)
  spline S168 degree 2 poles (21.3144, -16.8864) (21.4128, -16.9788) (21.662, -17.0809) (21.7775, -17.0809) knots 0 0 0 1 2 2 2
  spline S169 degree 2 poles (21.7775, -17.0809) (21.9428, -17.0809) (22.1118, -16.9435) (22.1118, -16.8305) knots 0 0 0 1 2 2 2
  spline S170 degree 2 poles (22.1118, -16.8305) (22.1118, -16.7405) (22.023, -16.6287) (21.927, -16.6007) knots 0 0 0 1 2 2 2
  spline S171 degree 2 poles (21.927, -16.6007) (21.8577, -16.5813) (21.7422, -16.5545) (21.6559, -16.5327) knots 0 0 0 1 2 2 2
  spline S172 degree 2 poles (21.6559, -16.5327) (21.5781, -16.512) (21.4554, -16.45) (21.408, -16.4002) knots 0 0 0 1 2 2 2
  spline S173 degree 2 poles (21.408, -16.4002) (21.3618, -16.3503) (21.3107, -16.2166) (21.3107, -16.1291) knots 0 0 0 1 2 2 2
  spline S174 degree 2 poles (21.3107, -16.1291) (21.3107, -15.9468) (21.5952, -15.7) (21.8152, -15.7) knots 0 0 0 1 2 2 2
  spline S175 degree 2 poles (21.8152, -15.7) (21.9416, -15.7) (22.1653, -15.7498) (22.2613, -15.7972) knots 0 0 0 1 2 2 2
  line L267 (22.2613, -15.7972) -> (22.2613, -16.0355)
  line L268 (22.2613, -16.0355) -> (22.2467, -16.0355)
  spline S176 degree 2 poles (22.2467, -16.0355) (22.175, -15.9699) (21.9513, -15.8726) (21.8285, -15.8726) knots 0 0 0 1 2 2 2
  spline S177 degree 2 poles (21.8285, -15.8726) (21.69, -15.8726) (21.5186, -16.0027) (21.5186, -16.1084) knots 0 0 0 1 2 2 2
  spline S178 degree 2 poles (21.5186, -16.1084) (21.5186, -16.2032) (21.6195, -16.3163) (21.7143, -16.3418) knots 0 0 0 1 2 2 2
  spline S179 degree 2 poles (21.7143, -16.3418) (21.7775, -16.3588) (21.961, -16.4026) (22.0218, -16.4208) knots 0 0 0 1 2 2 2
  spline S180 degree 2 poles (22.0218, -16.4208) (22.1762, -16.4682) (22.3196, -16.6591) (22.3196, -16.7989) knots 0 0 0 1 2 2 2
  spline S181 degree 2 poles (22.3196, -16.7989) (22.3196, -16.8876) (22.2479, -17.0578) (22.1835, -17.1173) knots 0 0 0 1 2 2 2
  spline S182 degree 2 poles (22.1835, -17.1173) (22.1118, -17.183) (21.9294, -17.2535) (21.7921, -17.2535) knots 0 0 0 1 2 2 2
  line L269 (8.0599, -15.8775) -> (7.3621, -15.8775)
  line L270 (7.3621, -15.8775) -> (7.3621, -16.3005)
  line L271 (7.3621, -16.3005) -> (8.0307, -16.3005)
  line L272 (8.0307, -16.3005) -> (8.0307, -16.478)
  line L273 (8.0307, -16.478) -> (7.3621, -16.478)
  line L274 (7.3621, -16.478) -> (7.3621, -17.2)
  line L275 (7.3621, -17.2) -> (7.1628, -17.2)
  line L276 (7.1628, -17.2) -> (7.1628, -15.7)
  line L277 (7.1628, -15.7) -> (8.0599, -15.7)
  line L278 (8.0599, -15.7) -> (8.0599, -15.8775)
  line L279 (8.0769, -17.2) -> (8.5826, -15.7)
  line L280 (8.5826, -15.7) -> (8.8281, -15.7)
  line L281 (8.8281, -15.7) -> (9.3338, -17.2)
  line L282 (9.3338, -17.2) -> (9.1235, -17.2)
  line L283 (9.1235, -17.2) -> (8.9873, -16.7806)
  line L284 (8.9873, -16.7806) -> (8.4148, -16.7806)
  line L285 (8.4148, -16.7806) -> (8.2787, -17.2)
  line L286 (8.2787, -17.2) -> (8.0769, -17.2)
  line L287 (8.9326, -16.6105) -> (8.7005, -15.9042)
  line L288 (8.7005, -15.9042) -> (8.4695, -16.6105)
  line L289 (8.4695, -16.6105) -> (8.9326, -16.6105)
  line L290 (9.9987, -17.2) -> (9.4177, -17.2)
  line L291 (9.4177, -17.2) -> (9.4177, -17.0468)
  line L292 (9.4177, -17.0468) -> (9.6085, -17.0468)
  line L293 (9.6085, -17.0468) -> (9.6085, -15.8532)
  line L294 (9.6085, -15.8532) -> (9.4177, -15.8532)
  line L295 (9.4177, -15.8532) -> (9.4177, -15.7)
  line L296 (9.4177, -15.7) -> (9.9987, -15.7)
  line L297 (9.9987, -15.7) -> (9.9987, -15.8532)
  line L298 (9.9987, -15.8532) -> (9.8078, -15.8532)
  line L299 (9.8078, -15.8532) -> (9.8078, -17.0468)
  line L300 (9.8078, -17.0468) -> (9.9987, -17.0468)
  line L301 (9.9987, -17.0468) -> (9.9987, -17.2)
  line L302 (11.1146, -17.2) -> (10.2454, -17.2)
  line L303 (10.2454, -17.2) -> (10.2454, -15.7)
  line L304 (10.2454, -15.7) -> (10.4448, -15.7)
  line L305 (10.4448, -15.7) -> (10.4448, -17.0225)
  line L306 (10.4448, -17.0225) -> (11.1146, -17.0225)
  line L307 (11.1146, -17.0225) -> (11.1146, -17.2)
  spline S183 degree 2 poles (-17.6371, 4.7319) (-17.7489, 4.7319) (-17.9325, 4.7988) (-17.9969, 4.8608) knots 0 0 0 1 2 2 2
  spline S184 degree 2 poles (-17.9969, 4.8608) (-18.0601, 4.9216) (-18.1258, 5.0869) (-18.1258, 5.1805) knots 0 0 0 1 2 2 2
  spline S185 degree 2 poles (-18.1258, 5.1805) (-18.1258, 5.302) (-17.9957, 5.5062) (-17.8717, 5.567) knots 0 0 0 1 2 2 2
  line L308 (-17.8717, 5.567) -> (-17.8717, 5.5731)
  spline S186 degree 2 poles (-17.8717, 5.5731) (-17.9823, 5.6375) (-18.0893, 5.7907) (-18.0893, 5.9049) knots 0 0 0 1 2 2 2
  spline S187 degree 2 poles (-18.0893, 5.9049) (-18.0893, 6.0739) (-17.834, 6.3) (-17.6371, 6.3) knots 0 0 0 1 2 2 2
  spline S188 degree 2 poles (-17.6371, 6.3) (-17.4329, 6.3) (-17.1861, 6.0861) (-17.1861, 5.9183) knots 0 0 0 1 2 2 2
  spline S189 degree 2 poles (-17.1861, 5.9183) (-17.1861, 5.8174) (-17.3041, 5.6205) (-17.4147, 5.5646) knots 0 0 0 1 2 2 2
  line L309 (-17.4147, 5.5646) -> (-17.4147, 5.5585)
  spline S190 degree 2 poles (-17.4147, 5.5585) (-17.2834, 5.4977) (-17.1485, 5.3227) (-17.1485, 5.1841) knots 0 0 0 1 2 2 2
  spline S191 degree 2 poles (-17.1485, 5.1841) (-17.1485, 4.9921) (-17.428, 4.7319) (-17.6371, 4.7319) knots 0 0 0 1 2 2 2
  spline S192 degree 2 poles (-17.3551, 5.1647) (-17.3551, 5.2571) (-17.428, 5.3665) (-17.5314, 5.4224) knots 0 0 0 1 2 2 2
  spline S193 degree 2 poles (-17.5314, 5.4224) (-17.5654, 5.4418) (-17.6797, 5.4868) (-17.7514, 5.516) knots 0 0 0 1 2 2 2
  spline S194 degree 2 poles (-17.7514, 5.516) (-17.834, 5.4613) (-17.9228, 5.2984) (-17.9228, 5.1951) knots 0 0 0 1 2 2 2
  spline S195 degree 2 poles (-17.9228, 5.1951) (-17.9228, 5.0589) (-17.7587, 4.8814) (-17.6347, 4.8814) knots 0 0 0 1 2 2 2
  spline S196 degree 2 poles (-17.6347, 4.8814) (-17.5083, 4.8814) (-17.3551, 5.0334) (-17.3551, 5.1647) knots 0 0 0 1 2 2 2